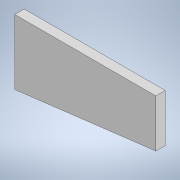
# Autodesk Inventor part: underDeckEastNearPool
Saved by Autodesk Inventor 2020.1 (Build 241239000, 239)
## iProperties
Created: 2019-08-11
Part Number: underDeckEastNearPool
Material: Generic
Document SubType Name: Modeling
Designer: steele
Density: 1 g/cm^3
Appearance: Default
Author: steele
Autodesk Inventor part; units mm, degrees
ref_plane "YZ Plane" through (0, 0, 0) normal (1, 0, 0) x (0, 1, 0)
ref_plane "XZ Plane" through (0, 0, 0) normal (0, 1, 0) x (-1, 0, 0)
ref_plane "XY Plane" through (0, 0, 0) normal (0, 0, 1) x (1, 0, 0)
sketch "Sketch1" plane through (0, 0, 0) normal (0, 0, 1) x (1, 0, 0)
  line L0 (0, 0) -> (0, 2108.7497)
  line L1 (0, 2108.7497) -> (4572, 2108.7497)
  line L2 (4572, 2108.7497) -> (4572, 559.8995)
  line L3 (0, 0) -> (4572, 559.8995)
  line L4 (2286, 2108.7497) -> (2286, 279.9497) construction
  dimension "d0" = 4572
  dimension "d1" = 1828.8
  dimension "d4" = 4606.1558
  dimension "d5" = 2108.7497
  dimension "d6" = 1548.8503
  constraints: 10 end point, 2 midpoint, 2 perpendicular, 1 vertical
  measures "d0" distance of L0.end L1.end
  measures "d1" distance of L4.start L4.end
  measures "d4" distance of L0.start L2.end
  measures "d5" distance of L0.end L0.start
  measures "d6" distance of L1.end L2.end
extrude "Extrusion1" add sketch "Sketch1" against normal blind 304.8
body "Solid1"
